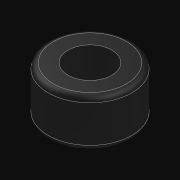
# Autodesk Inventor part: Spacer (Plastic)
Saved by Autodesk Inventor 2021.2 (Build 252289000, 289)
## iProperties
Created: 2020-04-19
Part Number: Spacer (Plastic)
Material: Acetal Resin, Black
Document SubType Name: Modeling
Designer: yuany
Density: 1.425 g/cm^3
Appearance: Smooth - Black
Author: yuany
Autodesk Inventor part; units mm, degrees
ref_plane "YZ Plane" through (0, 0, 0) normal (1, 0, 0) x (0, 1, 0)
ref_plane "XZ Plane" through (0, 0, 0) normal (0, 1, 0) x (-1, 0, 0)
ref_plane "XY Plane" through (0, 0, 0) normal (0, 0, 1) x (1, 0, 0)
sketch "Sketch1" plane through (0, 0, 0) normal (0, 1, 0) x (-1, 0, 0)
  circle A0 centre (5.2287, -5.6893) radius 4.064
  circle A1 centre (5.2287, -5.6893) radius 2.1209
  point P0 (0, 0)
  dimension "d0" = 8.128
  dimension "d1" = 4.2418
  constraints: 2 centre point, 1 coincident
  measures "d0" diameter of A0
  measures "d1" diameter of A1
extrude "Extrusion1" add sketch "Sketch1" along normal blind 4.6
fillet "Fillet1" radius 0.508 2 edges at (-1.1647, 4.6, -5.6893) (-1.1647, 0, -5.6893)
body "Solid1"
